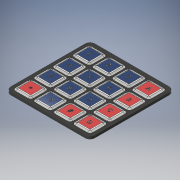
# Autodesk Inventor part: keypad
Saved by Autodesk Inventor 2019 (Build 230136000, 136)
## iProperties
Created: 2018-06-23
Part Number: keypad
Material: Generic
Document SubType Name: Modeling
Designer: Akshay
Density: 1 g/cm^3
Appearance: Default
Author: Akshay
Autodesk Inventor part; units mm, degrees
ref_plane "YZ Plane" through (0, 0, 0) normal (1, 0, 0) x (0, 1, 0)
ref_plane "XZ Plane" through (0, 0, 0) normal (0, 1, 0) x (-1, 0, 0)
ref_plane "XY Plane" through (0, 0, 0) normal (0, 0, 1) x (1, 0, 0)
sketch "Sketch1" plane through (0, 0, 0) normal (0, 1, 0) x (-1, 0, 0)
  line L0 (34, -34) -> (-34, -34)
  line L1 (-34, -34) -> (-34, 34)
  line L2 (-34, 34) -> (34, 34)
  line L3 (34, 34) -> (34, -34)
  line L4 (34, -34) -> (-34, 34) construction
  line L5 (-34, -34) -> (34, 34) construction
  point P0 (0, 0)
  dimension "d0" = 68
  dimension "d1" = 68
  constraints: 12 end point, 2 midpoint, 2 parallel, 1 horizontal, 1 perpendicular
  measures "d0" distance of L1.end L2.end
  measures "d1" distance of L0.end L1.end
extrude "Extrusion1" add sketch "Sketch1" along normal blind 2
fillet "Fillet1" radius 4 4 edges at (-34, 1, -34) (-34, 1, 34) (34, 1, 34) (34, 1, -34)
sketch "Sketch3" plane through (0, 2, 0) normal (0, 1, 0) x (1, 0, 0)
  line L0 (18, 29.4093) -> (30, 29.4093)
  line L1 (2, 29.4093) -> (14, 29.4093)
  line L2 (-30, 29.4093) -> (-18, 29.4093)
  line L3 (-14, 29.4093) -> (-2, 29.4093)
  line L4 (-30, 17.4093) -> (-30, 29.4093)
  line L5 (-18, 29.4093) -> (-18, 17.4093)
  line L6 (-14, 29.4093) -> (-14, 17.4093)
  line L7 (-18, 17.4093) -> (-30, 17.4093)
  line L8 (-2, 17.4093) -> (-14, 17.4093)
  line L9 (-2, 17.4093) -> (-2, 29.4093)
  line L10 (2, 29.4093) -> (2, 17.4093)
  line L11 (30, 17.4093) -> (18, 17.4093)
  line L12 (14, 17.4093) -> (2, 17.4093)
  line L13 (14, 17.4093) -> (14, 29.4093)
  line L14 (18, 29.4093) -> (18, 17.4093)
  line L15 (2, 13.4093) -> (14, 13.4093)
  line L16 (18, 13.4093) -> (30, 13.4093)
  line L17 (30, 1.9653) -> (18, 1.861)
  line L18 (18, 13.4093) -> (18, 1.861)
  line L19 (14, 1.8263) -> (14, 13.4093)
  line L20 (2, 13.4093) -> (2, 1.722)
  line L21 (-2, 1.6873) -> (-2, 13.4093)
  line L22 (-14, 13.4093) -> (-14, 1.5831)
  line L23 (-18, 13.4093) -> (-18, 1.5483)
  line L24 (-30, 1.4441) -> (-30, 13.4093)
  line L25 (-18, 1.5483) -> (-30, 1.4441)
  line L26 (-30, 13.4093) -> (-18, 13.4093)
  line L27 (-14, 13.4093) -> (-2, 13.4093)
  line L28 (14, 1.8263) -> (2, 1.722)
  line L29 (-2, 1.6873) -> (-14, 1.5831)
  line L30 (18, -2) -> (30, -2)
  line L31 (-30, -30) -> (-30, -18)
  line L32 (-30, -14) -> (-30, -2)
  line L33 (-18, -2) -> (-18, -14)
  line L34 (-18, -18) -> (-18, -30)
  line L35 (-30, -14) -> (-18, -14)
  line L36 (-30, -18) -> (-18, -18)
  line L37 (-14, -14) -> (-2, -14)
  line L38 (-14, -2) -> (-14, -14)
  line L39 (-14, -18) -> (-14, -30)
  line L40 (-2, -30) -> (-2, -18)
  line L41 (-2, -14) -> (-2, -2)
  line L42 (-14, -18) -> (-2, -18)
  line L43 (2, -14) -> (14, -14)
  line L44 (18, -14) -> (30, -14)
  line L45 (14, -30) -> (14, -18)
  line L46 (14, -14) -> (14, -2)
  line L47 (2, -2) -> (2, -14)
  line L48 (2, -18) -> (2, -30)
  line L49 (2, -18) -> (14, -18)
  line L50 (18, -18) -> (30, -18)
  line L51 (30, -30) -> (30, -18)
  line L52 (30, -14) -> (30, -2)
  line L53 (18, -2) -> (18, -14)
  line L54 (18, -18) -> (18, -30)
  line L55 (18, -30) -> (30, -30)
  line L56 (2, -30) -> (14, -30)
  line L57 (-30, -30) -> (-18, -30)
  line L58 (-14, -30) -> (-2, -30)
  line L59 (30, 1.9653) -> (30, 13.4093)
  line L60 (30, 17.4093) -> (30, 29.4093)
  line L61 (-30, -2) -> (-2, -2)
  line L62 (2, -2) -> (14, -2)
  point P0 (0, 0)
  point P1 (-34, -30)
  point P2 (-30, 34)
  constraints: 126 end point, 96 perpendicular, 4 horizontal, 2 point on line
extrude "Extrusion2" add sketch "Sketch3" along normal blind 1
fillet "Fillet2" radius 1 4 edges at (-30, 2.5, 18) (-18, 2.5, 18) (-30, 2.5, 30) (-18, 2.5, 30)
fillet "Fillet3" radius 1 4 edges at (-30, 2.5, 14) (-30, 2.5, 2) (-18, 2.5, 2) (-18, 2.5, 14)
fillet "Fillet4" radius 1 4 edges at (-18, 2.5, -1.5483) (-30, 2.5, -1.4441) (-18, 2.5, -13.4093) (-30, 2.5, -13.4093)
fillet "Fillet5" radius 1 4 edges at (-30, 2.5, -29.4093) (-18, 2.5, -29.4093) (-30, 2.5, -17.4093) (-18, 2.5, -17.4093)
fillet "Fillet6" radius 1 5 edges at (-14, 2.5, -17.4093) (-14, 2.5, -13.4093) (-14, 2.5, -29.4093) (-2, 2.5, -29.4093) (-2, 2.5, -17.4093)
fillet "Fillet7" radius 1 7 edges at (-2, 2.5, -13.4093) (-2, 2.5, -1.6873) (-14, 2.5, -1.5831) (-14, 2.5, 2) (-14, 2.5, 14) (-2, 2.5, 14) (-2, 2.5, 2)
fillet "Fillet8" radius 1 12 edges at (-2, 2.5, 18) (-2, 2.5, 30) (-14, 2.5, 30) (-14, 2.5, 18) (2, 2.5, 18) (2, 2.5, 30) (14, 2.5, 30) (14, 2.5, 18) (18, 2.5, 18) (30, 2.5, 30) (18, 2.5, 30) (30, 2.5, 18)
fillet "Fillet9" radius 1 8 edges at (2, 2.5, 2) (2, 2.5, 14) (14, 2.5, 14) (14, 2.5, 2) (18, 2.5, 14) (18, 2.5, 2) (30, 2.5, 2) (30, 2.5, 14)
fillet "Fillet10" radius 1 16 edges at (2, 2.5, -13.4093) (2, 2.5, -1.722) (14, 2.5, -1.8263) (14, 2.5, -13.4093) (18, 2.5, -13.4093) (18, 2.5, -1.861) (30, 2.5, -1.9653) (30, 2.5, -13.4093) (30, 2.5, -17.4093) (30, 2.5, -29.4093) (18, 2.5, -17.4093) (18, 2.5, -29.4093) (14, 2.5, -29.4093) (14, 2.5, -17.4093) (2, 2.5, -17.4093) (2, 2.5, -29.4093)
fillet "Fillet11" radius 1 8 edges at (-29.7071, 3, -17.7022) (-24, 3, -17.4093) (-18.2929, 3, -17.7022) (-18, 3, -23.4093) (-18.2929, 3, -29.1164) (-24, 3, -29.4093) (-29.7071, 3, -29.1164) (-30, 3, -23.4093)
fillet "Fillet12" radius 1 120 edges at (-13.7071, 3, -17.7022) (-8, 3, -17.4093) (-2.2929, 3, -17.7022) (-2, 3, -23.4093) (-2.2929, 3, -29.1164) (-8, 3, -29.4093) (-13.7071, 3, -29.1164) (-14, 3, -23.4093) (-13.704, 3, -1.8816) (-7.9913, 3, -1.6352) (-2.2898, 3, -1.9746) (-2, 3, -7.544) (-2.2929, 3, -13.1164) (-8, 3, -13.4093) (-13.7071, 3, -13.1164) (-14, 3, -7.5006) (-29.704, 3, -1.7426) (-23.9913, 3, -1.4963) (-18.2898, 3, -1.8356) (-18, 3, -7.4745) (-18.2929, 3, -13.1164) (-24, 3, -13.4093) (-29.7071, 3, -13.1164) (-30, 3, -7.4311) (2.296, 3, -2.0206) (8.0087, 3, -1.7742) (13.7102, 3, -2.1136) (14, 3, -7.6135) (13.7071, 3, -13.1164) (8, 3, -13.4093) (2.2929, 3, -13.1164) (2, 3, -7.57) (2.2929, 3, -17.7022) (8, 3, -17.4093) (13.7071, 3, -17.7022) (14, 3, -23.4093) (13.7071, 3, -29.1164) (8, 3, -29.4093) (2.2929, 3, -29.1164) (2, 3, -23.4093) (18.296, 3, -2.1596) (24.0087, 3, -1.9132) (29.7102, 3, -2.2526) (30, 3, -7.683) (29.7071, 3, -13.1164) (24, 3, -13.4093) (18.2929, 3, -13.1164) (18, 3, -7.6395) (18.2929, 3, -17.7022) (24, 3, -17.4093) (29.7071, 3, -17.7022) (30, 3, -23.4093) (29.7071, 3, -29.1164) (24, 3, -29.4093) (18.2929, 3, -29.1164) (18, 3, -23.4093) (18.2929, 3, 13.7071) (24, 3, 14) (29.7071, 3, 13.7071) (30, 3, 8) (29.7071, 3, 2.2929) (24, 3, 2) (18.2929, 3, 2.2929) (18, 3, 8) (18.2929, 3, 29.7071) (24, 3, 30) (29.7071, 3, 29.7071) (30, 3, 24) (29.7071, 3, 18.2929) (24, 3, 18) (18.2929, 3, 18.2929) (18, 3, 24) (2.2929, 3, 29.7071) (8, 3, 30) (13.7071, 3, 29.7071) (14, 3, 24) (13.7071, 3, 18.2929) (8, 3, 18) (2.2929, 3, 18.2929) (2, 3, 24) (2.2929, 3, 13.7071) (8, 3, 14) (13.7071, 3, 13.7071) (14, 3, 8) (13.7071, 3, 2.2929) (8, 3, 2) (2.2929, 3, 2.2929) (2, 3, 8) (-13.7071, 3, 29.7071) (-8, 3, 30) (-2.2929, 3, 29.7071) (-2, 3, 24) (-2.2929, 3, 18.2929) (-8, 3, 18) (-13.7071, 3, 18.2929) (-14, 3, 24) (-13.7071, 3, 13.7071) (-8, 3, 14) (-2.2929, 3, 13.7071) (-2, 3, 8) (-2.2929, 3, 2.2929) (-8, 3, 2) (-13.7071, 3, 2.2929) (-14, 3, 8) (-29.7071, 3, 13.7071) (-24, 3, 14) (-18.2929, 3, 13.7071) (-18, 3, 8) (-18.2929, 3, 2.2929) (-24, 3, 2) (-29.7071, 3, 2.2929) (-30, 3, 8) (-29.7071, 3, 29.7071) (-24, 3, 30) (-18.2929, 3, 29.7071) (-18, 3, 24) (-18.2929, 3, 18.2929) (-24, 3, 18) (-29.7071, 3, 18.2929) (-30, 3, 24)
fillet "Fillet13" radius 2 256 edges at (24, 2, 14) (24, 2.0005, 14) (29.7071, 2, 13.7071) (29.7071, 2.0005, 13.7071) (30, 2, 8) (30, 2.0005, 8) (29.7071, 2, 2.2929) (29.7071, 2.0005, 2.2929) (24, 2, 2) (24, 2.0005, 2) (18.2929, 2, 2.2929) (18.2929, 2.0005, 2.2929) (18, 2, 8) (18, 2.0005, 8) (18.2929, 2, 13.7071) (18.2929, 2.0005, 13.7071) (13.7071, 2, 13.7071) (13.7071, 2.0005, 13.7071) (8, 2, 14) (8, 2.0005, 14) (2.2929, 2, 13.7071) (2.2929, 2.0005, 13.7071) (2, 2, 8) (2, 2.0005, 8) (2.2929, 2, 2.2929) (2.2929, 2.0005, 2.2929) (8, 2, 2) (8, 2.0005, 2) (13.7071, 2, 2.2929) (13.7071, 2.0005, 2.2929) (14, 2, 8) (14, 2.0005, 8) (13.7071, 2, 29.7071) (13.7071, 2.0005, 29.7071) (8, 2, 30) (8, 2.0005, 30) (2.2929, 2, 29.7071) (2.2929, 2.0005, 29.7071) (2, 2, 24) (2, 2.0005, 24) (2.2929, 2, 18.2929) (2.2929, 2.0005, 18.2929) (8, 2, 18) (8, 2.0005, 18) (13.7071, 2, 18.2929) (13.7071, 2.0005, 18.2929) (14, 2, 24) (14, 2.0005, 24) (18.2929, 2, 18.2929) (18.2929, 2.0005, 18.2929) (24, 2, 18) (24, 2.0005, 18) (29.7071, 2, 18.2929) (29.7071, 2.0005, 18.2929) (30, 2, 24) (30, 2.0005, 24) (29.7071, 2, 29.7071) (29.7071, 2.0005, 29.7071) (24, 2, 30) (24, 2.0005, 30) (18.2929, 2, 29.7071) (18.2929, 2.0005, 29.7071) (18, 2, 24) (18, 2.0005, 24) (29.7102, 2, -2.2526) (29.7102, 2.0005, -2.2526) (24.0087, 2, -1.9132) (24.0087, 2.0005, -1.9132) (18.296, 2, -2.1596) (18.296, 2.0005, -2.1596) (18, 2, -7.6395) (18, 2.0005, -7.6395) (18.2929, 2, -13.1164) (18.2929, 2.0005, -13.1164) (24, 2, -13.4093) (24, 2.0005, -13.4093) (29.7071, 2, -13.1164) (29.7071, 2.0005, -13.1164) (30, 2, -7.683) (30, 2.0005, -7.683) (13.7102, 2, -2.1136) (13.7102, 2.0005, -2.1136) (8.0087, 2, -1.7742) (8.0087, 2.0005, -1.7742) (2.296, 2, -2.0206) (2.296, 2.0005, -2.0206) (2, 2, -7.57) (2, 2.0005, -7.57) (2.2929, 2, -13.1164) (2.2929, 2.0005, -13.1164) (8, 2, -13.4093) (8, 2.0005, -13.4093) (13.7071, 2, -13.1164) (13.7071, 2.0005, -13.1164) (14, 2, -7.6135) (14, 2.0005, -7.6135) (18.2929, 2, -29.1164) (18.2929, 2.0005, -29.1164) (24, 2, -29.4093) (24, 2.0005, -29.4093) (29.7071, 2, -29.1164) (29.7071, 2.0005, -29.1164) (30, 2.0005, -23.4093) (30, 2, -23.4093) (29.7071, 2.0005, -17.7022) (29.7071, 2, -17.7022) (24, 2, -17.4093) (24, 2.0005, -17.4093) (18.2929, 2, -17.7022) (18.2929, 2.0005, -17.7022) (18, 2, -23.4093) (18, 2.0005, -23.4093) (13.7071, 2, -17.7022) (13.7071, 2.0005, -17.7022) (8, 2, -17.4093) (8, 2.0005, -17.4093) (2.2929, 2, -17.7022) (2.2929, 2.0005, -17.7022) (2, 2, -23.4093) (2, 2.0005, -23.4093) (2.2929, 2, -29.1164) (2.2929, 2.0005, -29.1164) (8, 2, -29.4093) (8, 2.0005, -29.4093) (13.7071, 2, -29.1164) (13.7071, 2.0005, -29.1164) (14, 2, -23.4093) (14, 2.0005, -23.4093) (-2.2929, 2, -17.7022) (-2.2929, 2.0005, -17.7022) (-8, 2, -17.4093) (-8, 2.0005, -17.4093) (-13.7071, 2, -17.7022) (-13.7071, 2.0005, -17.7022) (-14, 2, -23.4093) (-14, 2.0005, -23.4093) (-13.7071, 2, -29.1164) (-13.7071, 2.0005, -29.1164) (-8, 2, -29.4093) (-8, 2.0005, -29.4093) (-2.2929, 2, -29.1164) (-2.2929, 2.0005, -29.1164) (-2, 2, -23.4093) (-2, 2.0005, -23.4093) (-2.2898, 2, -1.9746) (-2.2898, 2.0005, -1.9746) (-7.9913, 2, -1.6352) (-7.9913, 2.0005, -1.6352) (-13.704, 2, -1.8816) (-13.704, 2.0005, -1.8816) (-14, 2, -7.5006) (-14, 2.0005, -7.5006) (-13.7071, 2, -13.1164) (-13.7071, 2.0005, -13.1164) (-8, 2, -13.4093) (-8, 2.0005, -13.4093) (-2.2929, 2, -13.1164) (-2.2929, 2.0005, -13.1164) (-2, 2, -7.544) (-2, 2.0005, -7.544) (-2.2929, 2, 13.7071) (-2.2929, 2.0005, 13.7071) (-8, 2, 14) (-8, 2.0005, 14) (-13.7071, 2, 13.7071) (-13.7071, 2.0005, 13.7071) (-14, 2, 8) (-14, 2.0005, 8) (-13.7071, 2, 2.2929) (-13.7071, 2.0005, 2.2929) (-8, 2, 2) (-8, 2.0005, 2) (-2.2929, 2, 2.2929) (-2.2929, 2.0005, 2.2929) (-2, 2, 8) (-2, 2.0005, 8) (-2.2929, 2, 29.7071) (-2.2929, 2.0005, 29.7071) (-8, 2, 30) (-8, 2.0005, 30) (-13.7071, 2, 29.7071) (-13.7071, 2.0005, 29.7071) (-14, 2, 24) (-14, 2.0005, 24) (-13.7071, 2, 18.2929) (-13.7071, 2.0005, 18.2929) (-8, 2, 18) (-8, 2.0005, 18) (-2.2929, 2, 18.2929) (-2.2929, 2.0005, 18.2929) (-2, 2, 24) (-2, 2.0005, 24) (-18.2929, 2, 29.7071) (-18.2929, 2.0005, 29.7071) (-24, 2, 30) (-24, 2.0005, 30) (-29.7071, 2, 29.7071) (-29.7071, 2.0005, 29.7071) (-30, 2, 24) (-30, 2.0005, 24) (-29.7071, 2, 18.2929) (-29.7071, 2.0005, 18.2929) (-24, 2, 18) (-24, 2.0005, 18) (-18.2929, 2, 18.2929) (-18.2929, 2.0005, 18.2929) (-18, 2, 24) (-18, 2.0005, 24) (-18.2929, 2, 13.7071) (-18.2929, 2.0005, 13.7071) (-24, 2, 14) (-24, 2.0005, 14) (-29.7071, 2, 13.7071) (-29.7071, 2.0005, 13.7071) (-30, 2, 8) (-30, 2.0005, 8) (-29.7071, 2, 2.2929) (-29.7071, 2.0005, 2.2929) (-24, 2, 2) (-24, 2.0005, 2) (-18.2929, 2, 2.2929) (-18.2929, 2.0005, 2.2929) (-18, 2, 8) (-18, 2.0005, 8) (-18.2898, 2, -1.8356) (-18.2898, 2.0005, -1.8356) (-23.9913, 2, -1.4963) (-23.9913, 2.0005, -1.4963) (-29.704, 2, -1.7426) (-29.704, 2.0005, -1.7426) (-30, 2, -7.4311) (-30, 2.0005, -7.4311) (-29.7071, 2, -13.1164) (-29.7071, 2.0005, -13.1164) (-24, 2, -13.4093) (-24, 2.0005, -13.4093) (-18.2929, 2, -13.1164) (-18.2929, 2.0005, -13.1164) (-18, 2, -7.4745) (-18, 2.0005, -7.4745) (-18.2929, 2, -17.7022) (-18.2929, 2.0005, -17.7022) (-24, 2, -17.4093) (-24, 2.0005, -17.4093) (-29.7071, 2, -17.7022) (-29.7071, 2.0005, -17.7022) (-30, 2, -23.4093) (-30, 2.0005, -23.4093) (-29.7071, 2, -29.1164) (-29.7071, 2.0005, -29.1164) (-24, 2, -29.4093) (-24, 2.0005, -29.4093) (-18.2929, 2, -29.1164) (-18.2929, 2.0005, -29.1164) (-18, 2, -23.4093) (-18, 2.0005, -23.4093)
sketch "Sketch4" plane through (0, 3, 0) normal (0, 1, 0) x (1, 0, 0)
  line L0 (-25.4936, 25.6237) -> (-19.6405, 25.6237) construction
  line L1 (-19.6405, 25.6237) -> (-19.6405, 19.1202) construction
  line L2 (-19.6405, 19.1202) -> (-25.4936, 19.1202) construction
  line L3 (-25.4936, 19.1202) -> (-25.4936, 25.6237) construction
  line L4 (-9.6251, 25.2335) -> (-7.3379, 25.2335) construction
  line L5 (-7.3379, 25.2335) -> (-7.3379, 22.1213) construction
  line L6 (-7.3379, 22.1213) -> (-9.6251, 22.1213) construction
  line L7 (-9.6251, 22.1213) -> (-9.6251, 25.2335) construction
  line L8 (6.3734, 24.9733) -> (8.6606, 24.9733) construction
  line L9 (8.6606, 24.9733) -> (8.6606, 21.7969) construction
  line L10 (8.6606, 21.7969) -> (6.3734, 21.7969) construction
  line L11 (6.3734, 21.7969) -> (6.3734, 24.9733) construction
  line L12 (-24.9733, 8.9748) -> (-22.426, 8.9748) construction
  line L13 (-22.426, 8.9748) -> (-22.426, 5.9268) construction
  line L14 (-22.426, 5.9268) -> (-24.9733, 5.9268) construction
  line L15 (-24.9733, 5.9268) -> (-24.9733, 8.9748) construction
  line L16 (-8.9748, 8.8447) -> (-6.6876, 8.8447) construction
  line L17 (-6.6876, 8.8447) -> (-6.6876, 5.7325) construction
  line L18 (-6.6876, 5.7325) -> (-8.9748, 5.7325) construction
  line L19 (-8.9748, 5.7325) -> (-8.9748, 8.8447) construction
  line L20 (6.7636, 9.365) -> (9.0508, 9.365) construction
  line L21 (9.0508, 9.365) -> (9.0508, 6.196) construction
  line L22 (9.0508, 6.196) -> (6.7636, 6.196) construction
  line L23 (6.7636, 6.196) -> (6.7636, 9.365) construction
  line L24 (-25.4395, -6.3515) -> (-23.1523, -6.3515) construction
  line L25 (-23.1523, -6.3515) -> (-23.1523, -9.3995) construction
  line L26 (-23.1523, -9.3995) -> (-25.4395, -9.3995) construction
  line L27 (-25.4395, -9.3995) -> (-25.4395, -6.3515) construction
  line L28 (-9.2349, -6.6335) -> (-6.9477, -6.6335) construction
  line L29 (-6.9477, -6.6335) -> (-6.9477, -9.8199) construction
  line L30 (-6.9477, -9.8199) -> (-9.2349, -9.8199) construction
  line L31 (-9.2349, -9.8199) -> (-9.2349, -6.6335) construction
  line L32 (6.8094, -6.4337) -> (8.9208, -6.4337) construction
  line L33 (8.9208, -6.4337) -> (8.9208, -9.6027) construction
  line L34 (8.9208, -9.6027) -> (6.8094, -9.6027) construction
  line L35 (6.8094, -9.6027) -> (6.8094, -6.4337) construction
  line L36 (-8.7057, -22.502) -> (-6.4185, -22.502) construction
  line L37 (-6.4185, -22.502) -> (-6.4185, -25.676) construction
  line L38 (-6.4185, -25.676) -> (-8.7057, -25.676) construction
  line L39 (-8.7057, -25.676) -> (-8.7057, -22.502) construction
  line L40 (23.0223, 24.8433) -> (25.5763, 24.8433) construction
  line L41 (25.5763, 24.8433) -> (25.5763, 21.7953) construction
  line L42 (25.5763, 21.7953) -> (23.0223, 21.7953) construction
  line L43 (23.0223, 21.7953) -> (23.0223, 24.8433) construction
  line L44 (22.7622, 9.2349) -> (26.2727, 9.2349) construction
  line L45 (26.2727, 9.2349) -> (26.2727, 6.1869) construction
  line L46 (26.2727, 6.1869) -> (22.7622, 6.1869) construction
  line L47 (22.7622, 6.1869) -> (22.7622, 9.2349) construction
  line L48 (22.3719, -5.9832) -> (24.8889, -5.9832) construction
  line L49 (24.8889, -5.9832) -> (24.8889, -9.1399) construction
  line L50 (24.8889, -9.1399) -> (22.3719, -9.1399) construction
  line L51 (22.3719, -9.1399) -> (22.3719, -5.9832) construction
  line L52 (22.3719, -22.502) -> (25.2149, -22.502) construction
  line L53 (25.2149, -22.502) -> (25.2149, -25.55) construction
  line L54 (25.2149, -25.55) -> (22.3719, -25.55) construction
  line L55 (22.3719, -25.55) -> (22.3719, -22.502) construction
  line L56 (-25.1536, -22.9863) -> (-22.8664, -22.9863) construction
  line L57 (-22.8664, -22.9863) -> (-22.8664, -24.8808) construction
  line L58 (-22.8664, -24.8808) -> (-25.1536, -24.8808) construction
  line L59 (-25.1536, -24.8808) -> (-25.1536, -22.9863) construction
  line L60 (6.5254, -22.296) -> (9.5758, -22.296) construction
  line L61 (9.5758, -22.296) -> (9.5758, -25.344) construction
  line L62 (9.5758, -25.344) -> (6.5254, -25.344) construction
  line L63 (6.5254, -25.344) -> (6.5254, -22.296) construction
  line L64 (23.0025, 21.7953) -> (24.0301, 24.8433)
  line L65 (24.0301, 24.8433) -> (24.529, 24.8433)
  line L66 (24.529, 24.8433) -> (25.5565, 21.7953)
  line L67 (25.5565, 21.7953) -> (25.1292, 21.7953)
  line L68 (25.1292, 21.7953) -> (24.8526, 22.6474)
  line L69 (24.8526, 22.6474) -> (23.6892, 22.6474)
  line L70 (23.6892, 22.6474) -> (23.4126, 21.7953)
  line L71 (23.4126, 21.7953) -> (23.0025, 21.7953)
  line L72 (24.7414, 22.9932) -> (24.2697, 24.4283)
  line L73 (24.2697, 24.4283) -> (23.8004, 22.9932)
  line L74 (23.8004, 22.9932) -> (24.7414, 22.9932)
  spline S0 degree 2 poles (7.4182, 24.6201) (7.3071, 24.6201) (7.0872, 24.5658) (6.981, 24.5238) knots 0 0 0 1 2 2 2
  spline S1 degree 2 poles (6.981, 24.5238) (6.8822, 24.4818) (6.7365, 24.3929) (6.6797, 24.3534) knots 0 0 0 1 2 2 2
  line L75 (6.6797, 24.3534) -> (6.655, 24.3534)
  line L76 (6.655, 24.3534) -> (6.655, 24.7856)
  spline S2 degree 2 poles (6.655, 24.7856) (6.7884, 24.8573) (7.2453, 24.9733) (7.4503, 24.9733) knots 0 0 0 1 2 2 2
  spline S3 degree 2 poles (7.4503, 24.9733) (7.6578, 24.9733) (7.9666, 24.8894) (8.0925, 24.8004) knots 0 0 0 1 2 2 2
  spline S4 degree 2 poles (8.0925, 24.8004) (8.2259, 24.7041) (8.3642, 24.425) (8.3642, 24.2373) knots 0 0 0 1 2 2 2
  spline S5 degree 2 poles (8.3642, 24.2373) (8.3642, 23.9853) (8.0333, 23.605) (7.8011, 23.5556) knots 0 0 0 1 2 2 2
  line L77 (7.8011, 23.5556) -> (7.8011, 23.5259)
  spline S6 degree 2 poles (7.8011, 23.5259) (7.8974, 23.5062) (8.1172, 23.4172) (8.2111, 23.3283) knots 0 0 0 1 2 2 2
  spline S7 degree 2 poles (8.2111, 23.3283) (8.305, 23.2419) (8.4235, 22.9652) (8.4235, 22.7651) knots 0 0 0 1 2 2 2
  spline S8 degree 2 poles (8.4235, 22.7651) (8.4235, 22.5601) (8.2827, 22.2119) (8.1543, 22.0785) knots 0 0 0 1 2 2 2
  spline S9 degree 2 poles (8.1543, 22.0785) (8.0209, 21.9402) (7.643, 21.7969) (7.4034, 21.7969) knots 0 0 0 1 2 2 2
  spline S10 degree 2 poles (7.4034, 21.7969) (7.1737, 21.7969) (6.7241, 21.9081) (6.571, 21.9846) knots 0 0 0 1 2 2 2
  line L78 (6.571, 21.9846) -> (6.571, 22.4169)
  line L79 (6.571, 22.4169) -> (6.6006, 22.4169)
  spline S11 degree 2 poles (6.6006, 22.4169) (6.7291, 22.323) (7.1638, 22.1501) (7.3787, 22.1501) knots 0 0 0 1 2 2 2
  spline S12 degree 2 poles (7.3787, 22.1501) (7.5047, 22.1501) (7.7566, 22.2292) (7.8406, 22.3205) knots 0 0 0 1 2 2 2
  spline S13 degree 2 poles (7.8406, 22.3205) (7.9221, 22.4119) (8.0086, 22.6293) (8.0086, 22.7948) knots 0 0 0 1 2 2 2
  spline S14 degree 2 poles (8.0086, 22.7948) (8.0086, 22.9603) (7.9122, 23.1752) (7.8258, 23.2369) knots 0 0 0 1 2 2 2
  spline S15 degree 2 poles (7.8258, 23.2369) (7.7393, 23.2987) (7.5047, 23.3456) (7.3664, 23.3456) knots 0 0 0 1 2 2 2
  line L80 (7.3664, 23.3456) -> (7.1934, 23.3456)
  line L81 (7.1934, 23.3456) -> (7.1934, 23.684)
  line L82 (7.1934, 23.684) -> (7.3293, 23.684)
  spline S16 degree 2 poles (7.3293, 23.684) (7.6035, 23.684) (7.9493, 23.9458) (7.9493, 24.1953) knots 0 0 0 1 2 2 2
  spline S17 degree 2 poles (7.9493, 24.1953) (7.9493, 24.3114) (7.8604, 24.4769) (7.7887, 24.5263) knots 0 0 0 1 2 2 2
  spline S18 degree 2 poles (7.7887, 24.5263) (7.7122, 24.5781) (7.5244, 24.6201) (7.4182, 24.6201) knots 0 0 0 1 2 2 2
  line L83 (-7.5232, 22.1213) -> (-9.4028, 22.1213)
  line L84 (-9.4028, 22.1213) -> (-9.4028, 22.5535)
  spline S19 degree 2 poles (-9.4028, 22.5535) (-9.2003, 22.7437) (-8.8397, 23.0969) (-8.6668, 23.2871) knots 0 0 0 1 2 2 2
  spline S20 degree 2 poles (-8.6668, 23.2871) (-8.3185, 23.67) (-8.0641, 24.1294) (-8.0641, 24.3739) knots 0 0 0 1 2 2 2
  spline S21 degree 2 poles (-8.0641, 24.3739) (-8.0641, 24.5024) (-8.1431, 24.695) (-8.2148, 24.7568) knots 0 0 0 1 2 2 2
  spline S22 degree 2 poles (-8.2148, 24.7568) (-8.2864, 24.8185) (-8.4741, 24.8803) (-8.5877, 24.8803) knots 0 0 0 1 2 2 2
  spline S23 degree 2 poles (-8.5877, 24.8803) (-8.6964, 24.8803) (-8.9187, 24.8259) (-9.02, 24.7839) knots 0 0 0 1 2 2 2
  spline S24 degree 2 poles (-9.02, 24.7839) (-9.1064, 24.7494) (-9.267, 24.6506) (-9.3164, 24.616) knots 0 0 0 1 2 2 2
  line L85 (-9.3164, 24.616) -> (-9.3386, 24.616)
  line L86 (-9.3386, 24.616) -> (-9.3386, 25.0507)
  spline S25 degree 2 poles (-9.3386, 25.0507) (-9.2126, 25.1125) (-8.7606, 25.2335) (-8.5581, 25.2335) knots 0 0 0 1 2 2 2
  spline S26 degree 2 poles (-8.5581, 25.2335) (-8.1308, 25.2335) (-7.6491, 24.7815) (-7.6491, 24.3961) knots 0 0 0 1 2 2 2
  spline S27 degree 2 poles (-7.6491, 24.3961) (-7.6491, 24.2158) (-7.7331, 23.9145) (-7.8072, 23.7861) knots 0 0 0 1 2 2 2
  spline S28 degree 2 poles (-7.8072, 23.7861) (-7.8813, 23.6527) (-8.0962, 23.3908) (-8.2148, 23.2649) knots 0 0 0 1 2 2 2
  spline S29 degree 2 poles (-8.2148, 23.2649) (-8.4074, 23.0549) (-8.8792, 22.6054) (-9.02, 22.4745) knots 0 0 0 1 2 2 2
  line L87 (-9.02, 22.4745) -> (-7.5232, 22.4745)
  line L88 (-7.5232, 22.4745) -> (-7.5232, 22.1213)
  line L89 (-23.5448, 22.5658) -> (-25.0317, 22.5658)
  line L90 (-25.0317, 22.5658) -> (-25.0317, 22.877)
  line L91 (-25.0317, 22.877) -> (-24.4784, 22.877)
  line L92 (-24.4784, 22.877) -> (-24.4784, 24.9197)
  line L93 (-24.4784, 24.9197) -> (-25.0317, 24.9197)
  line L94 (-25.0317, 24.9197) -> (-25.0317, 25.1988)
  spline S30 degree 2 poles (-25.0317, 25.1988) (-24.718, 25.1988) (-24.4216, 25.3767) (-24.4019, 25.6237) knots 0 0 0 1 2 2 2
  line L95 (-24.4019, 25.6237) -> (-24.0857, 25.6237)
  line L96 (-24.0857, 25.6237) -> (-24.0857, 22.877)
  line L97 (-24.0857, 22.877) -> (-23.5448, 22.877)
  line L98 (-23.5448, 22.877) -> (-23.5448, 22.5658)
  line L99 (-22.7898, 6.9741) -> (-23.1529, 6.9741)
  line L100 (-23.1529, 6.9741) -> (-23.1529, 5.9268)
  line L101 (-23.1529, 5.9268) -> (-23.5457, 5.9268)
  line L102 (-23.5457, 5.9268) -> (-23.5457, 6.9741)
  line L103 (-23.5457, 6.9741) -> (-24.8918, 6.9741)
  line L104 (-24.8918, 6.9741) -> (-24.8918, 7.4039)
  line L105 (-24.8918, 7.4039) -> (-23.5284, 8.9748)
  line L106 (-23.5284, 8.9748) -> (-23.1529, 8.9748)
  line L107 (-23.1529, 8.9748) -> (-23.1529, 7.3026)
  line L108 (-23.1529, 7.3026) -> (-22.7898, 7.3026)
  line L109 (-22.7898, 7.3026) -> (-22.7898, 6.9741)
  line L110 (-23.5457, 7.3026) -> (-23.5457, 8.4931)
  line L111 (-23.5457, 8.4931) -> (-24.5707, 7.3026)
  line L112 (-24.5707, 7.3026) -> (-23.5457, 7.3026)
  line L113 (-23.303, -6.8085) -> (-24.622, -9.3995)
  line L114 (-24.622, -9.3995) -> (-25.0567, -9.3995)
  line L115 (-25.0567, -9.3995) -> (-23.6636, -6.7097)
  line L116 (-23.6636, -6.7097) -> (-25.237, -6.7097)
  line L117 (-25.237, -6.7097) -> (-25.237, -6.3515)
  line L118 (-25.237, -6.3515) -> (-23.303, -6.3515)
  line L119 (-23.303, -6.3515) -> (-23.303, -6.8085)
  line L120 (-23.0911, -24.3547) -> (-23.2245, -24.5795)
  line L121 (-23.2245, -24.5795) -> (-23.8939, -24.1349)
  line L122 (-23.8939, -24.1349) -> (-23.8791, -24.8808)
  line L123 (-23.8791, -24.8808) -> (-24.1359, -24.8808)
  line L124 (-24.1359, -24.8808) -> (-24.1236, -24.1349)
  line L125 (-24.1236, -24.1349) -> (-24.788, -24.582)
  line L126 (-24.788, -24.582) -> (-24.9239, -24.3572)
  line L127 (-24.9239, -24.3572) -> (-24.2002, -23.9324)
  line L128 (-24.2002, -23.9324) -> (-24.9239, -23.51)
  line L129 (-24.9239, -23.51) -> (-24.788, -23.2852)
  line L130 (-24.788, -23.2852) -> (-24.1211, -23.7323)
  line L131 (-24.1211, -23.7323) -> (-24.1359, -22.9863)
  line L132 (-24.1359, -22.9863) -> (-23.8791, -22.9863)
  line L133 (-23.8791, -22.9863) -> (-23.8964, -23.7323)
  line L134 (-23.8964, -23.7323) -> (-23.2245, -23.2877)
  line L135 (-23.2245, -23.2877) -> (-23.0911, -23.5125)
  line L136 (-23.0911, -23.5125) -> (-23.8148, -23.9324)
  line L137 (-23.8148, -23.9324) -> (-23.0911, -24.3547)
  spline S31 degree 2 poles (-6.9049, 6.765) (-6.9049, 6.5451) (-7.0457, 6.1697) (-7.1742, 6.0314) knots 0 0 0 1 2 2 2
  spline S32 degree 2 poles (-7.1742, 6.0314) (-7.3026, 5.8931) (-7.6854, 5.7325) (-7.9226, 5.7325) knots 0 0 0 1 2 2 2
  spline S33 degree 2 poles (-7.9226, 5.7325) (-8.1399, 5.7325) (-8.5648, 5.8288) (-8.7204, 5.9054) knots 0 0 0 1 2 2 2
  line L138 (-8.7204, 5.9054) -> (-8.7204, 6.3377)
  line L139 (-8.7204, 6.3377) -> (-8.6907, 6.3377)
  spline S34 degree 2 poles (-8.6907, 6.3377) (-8.6438, 6.3031) (-8.4684, 6.2142) (-8.3622, 6.1746) knots 0 0 0 1 2 2 2
  spline S35 degree 2 poles (-8.3622, 6.1746) (-8.2412, 6.1326) (-8.0411, 6.0857) (-7.9152, 6.0857) knots 0 0 0 1 2 2 2
  spline S36 degree 2 poles (-7.9152, 6.0857) (-7.7917, 6.0857) (-7.5595, 6.1746) (-7.4755, 6.271) knots 0 0 0 1 2 2 2
  spline S37 degree 2 poles (-7.4755, 6.271) (-7.3989, 6.3624) (-7.3199, 6.6044) (-7.3199, 6.7674) knots 0 0 0 1 2 2 2
  spline S38 degree 2 poles (-7.3199, 6.7674) (-7.3199, 6.9305) (-7.4088, 7.1379) (-7.4928, 7.2071) knots 0 0 0 1 2 2 2
  spline S39 degree 2 poles (-7.4928, 7.2071) (-7.5792, 7.2837) (-7.8361, 7.3479) (-7.9917, 7.3479) knots 0 0 0 1 2 2 2
  spline S40 degree 2 poles (-7.9917, 7.3479) (-8.1597, 7.3479) (-8.4931, 7.296) (-8.5944, 7.2738) knots 0 0 0 1 2 2 2
  line L140 (-8.5944, 7.2738) -> (-8.5944, 8.8447)
  line L141 (-8.5944, 8.8447) -> (-6.9222, 8.8447)
  line L142 (-6.9222, 8.8447) -> (-6.9222, 8.4866)
  line L143 (-6.9222, 8.4866) -> (-8.2017, 8.4866)
  line L144 (-8.2017, 8.4866) -> (-8.2017, 7.6739)
  spline S41 degree 2 poles (-8.2017, 7.6739) (-8.1276, 7.6838) (-7.9843, 7.6912) (-7.925, 7.6912) knots 0 0 0 1 2 2 2
  spline S42 degree 2 poles (-7.925, 7.6912) (-7.6904, 7.6912) (-7.3668, 7.6147) (-7.2186, 7.501) knots 0 0 0 1 2 2 2
  spline S43 degree 2 poles (-7.2186, 7.501) (-7.0679, 7.3874) (-6.9049, 7.0416) (-6.9049, 6.765) knots 0 0 0 1 2 2 2
  spline S44 degree 2 poles (-8.0913, -9.8199) (-8.3186, -9.8199) (-8.6915, -9.684) (-8.8224, -9.558) knots 0 0 0 1 2 2 2
  spline S45 degree 2 poles (-8.8224, -9.558) (-8.9509, -9.4345) (-9.0843, -9.0986) (-9.0843, -8.9084) knots 0 0 0 1 2 2 2
  spline S46 degree 2 poles (-9.0843, -8.9084) (-9.0843, -8.6614) (-8.82, -8.2465) (-8.568, -8.123) knots 0 0 0 1 2 2 2
  line L145 (-8.568, -8.123) -> (-8.568, -8.1106)
  spline S47 degree 2 poles (-8.568, -8.1106) (-8.7928, -7.9797) (-9.0102, -7.6685) (-9.0102, -7.4363) knots 0 0 0 1 2 2 2
  spline S48 degree 2 poles (-9.0102, -7.4363) (-9.0102, -7.093) (-8.4915, -6.6335) (-8.0913, -6.6335) knots 0 0 0 1 2 2 2
  spline S49 degree 2 poles (-8.0913, -6.6335) (-7.6764, -6.6335) (-7.1749, -7.0683) (-7.1749, -7.4091) knots 0 0 0 1 2 2 2
  spline S50 degree 2 poles (-7.1749, -7.4091) (-7.1749, -7.6141) (-7.4145, -8.0143) (-7.6393, -8.1279) knots 0 0 0 1 2 2 2
  line L146 (-7.6393, -8.1279) -> (-7.6393, -8.1403)
  spline S51 degree 2 poles (-7.6393, -8.1403) (-7.3725, -8.2638) (-7.0984, -8.6194) (-7.0984, -8.901) knots 0 0 0 1 2 2 2
  spline S52 degree 2 poles (-7.0984, -8.901) (-7.0984, -9.2913) (-7.6665, -9.8199) (-8.0913, -9.8199) knots 0 0 0 1 2 2 2
  spline S53 degree 2 poles (-7.5183, -8.9405) (-7.5183, -8.7528) (-7.6665, -8.5305) (-7.8764, -8.4169) knots 0 0 0 1 2 2 2
  spline S54 degree 2 poles (-7.8764, -8.4169) (-7.9456, -8.3774) (-8.1778, -8.286) (-8.3235, -8.2267) knots 0 0 0 1 2 2 2
  spline S55 degree 2 poles (-8.3235, -8.2267) (-8.4915, -8.3379) (-8.6718, -8.6688) (-8.6718, -8.8788) knots 0 0 0 1 2 2 2
  spline S56 degree 2 poles (-8.6718, -8.8788) (-8.6718, -9.1554) (-8.3383, -9.5161) (-8.0864, -9.5161) knots 0 0 0 1 2 2 2
  spline S57 degree 2 poles (-8.0864, -9.5161) (-7.8295, -9.5161) (-7.5183, -9.2073) (-7.5183, -8.9405) knots 0 0 0 1 2 2 2
  spline S58 degree 2 poles (-7.5751, -7.4141) (-7.5751, -7.2091) (-7.8493, -6.9349) (-8.0938, -6.9349) knots 0 0 0 1 2 2 2
  spline S59 degree 2 poles (-8.0938, -6.9349) (-8.3161, -6.9349) (-8.6001, -7.1794) (-8.6001, -7.3894) knots 0 0 0 1 2 2 2
  spline S60 degree 2 poles (-8.6001, -7.3894) (-8.6001, -7.54) (-8.4544, -7.75) (-8.3087, -7.834) knots 0 0 0 1 2 2 2
  spline S61 degree 2 poles (-8.3087, -7.834) (-8.2469, -7.8686) (-7.9851, -7.9896) (-7.8789, -8.0242) knots 0 0 0 1 2 2 2
  spline S62 degree 2 poles (-7.8789, -8.0242) (-7.7011, -7.8883) (-7.5751, -7.5993) (-7.5751, -7.4141) knots 0 0 0 1 2 2 2
  spline S63 degree 2 poles (-6.5864, -24.0878) (-6.5864, -24.9078) (-7.0631, -25.676) (-7.5596, -25.676) knots 0 0 0 1 2 2 2
  spline S64 degree 2 poles (-7.5596, -25.676) (-8.0635, -25.676) (-8.5353, -24.893) (-8.5353, -24.0902) knots 0 0 0 1 2 2 2
  spline S65 degree 2 poles (-8.5353, -24.0902) (-8.5353, -23.2653) (-8.0586, -22.502) (-7.5596, -22.502) knots 0 0 0 1 2 2 2
  spline S66 degree 2 poles (-7.5596, -22.502) (-7.0582, -22.502) (-6.5864, -23.2924) (-6.5864, -24.0878) knots 0 0 0 1 2 2 2
  spline S67 degree 2 poles (-7.1101, -25.0165) (-7.0508, -24.8658) (-7.0014, -24.4015) (-7.0014, -24.0878) knots 0 0 0 1 2 2 2
  spline S68 degree 2 poles (-7.0014, -24.0878) (-7.0014, -23.7741) (-7.0508, -23.3122) (-7.1125, -23.1566) knots 0 0 0 1 2 2 2
  spline S69 degree 2 poles (-7.1125, -23.1566) (-7.1743, -23.001) (-7.3892, -22.8404) (-7.5596, -22.8404) knots 0 0 0 1 2 2 2
  spline S70 degree 2 poles (-7.5596, -22.8404) (-7.73, -22.8404) (-7.9499, -23.001) (-8.0141, -23.1615) knots 0 0 0 1 2 2 2
  spline S71 degree 2 poles (-8.0141, -23.1615) (-8.0759, -23.3171) (-8.1203, -23.7914) (-8.1203, -24.0902) knots 0 0 0 1 2 2 2
  spline S72 degree 2 poles (-8.1203, -24.0902) (-8.1203, -24.4113) (-8.0808, -24.8411) (-8.0166, -25.0091) knots 0 0 0 1 2 2 2
  spline S73 degree 2 poles (-8.0166, -25.0091) (-7.9573, -25.1672) (-7.7375, -25.3376) (-7.5596, -25.3376) knots 0 0 0 1 2 2 2
  spline S74 degree 2 poles (-7.5596, -25.3376) (-7.3917, -25.3376) (-7.1718, -25.177) (-7.1101, -25.0165) knots 0 0 0 1 2 2 2
  spline S75 degree 2 poles (6.9477, -7.4859) (6.9477, -7.2513) (7.1009, -6.861) (7.2342, -6.7202) knots 0 0 0 1 2 2 2
  spline S76 degree 2 poles (7.2342, -6.7202) (7.3602, -6.5844) (7.7282, -6.4337) (7.916, -6.4337) knots 0 0 0 1 2 2 2
  spline S77 degree 2 poles (7.916, -6.4337) (8.1259, -6.4337) (8.4668, -6.5745) (8.5927, -6.7079) knots 0 0 0 1 2 2 2
  spline S78 degree 2 poles (8.5927, -6.7079) (8.7508, -6.8758) (8.9237, -7.4192) (8.9237, -7.8367) knots 0 0 0 1 2 2 2
  spline S79 degree 2 poles (8.9237, -7.8367) (8.9237, -8.2146) (8.7533, -8.8914) (8.5878, -9.1161) knots 0 0 0 1 2 2 2
  spline S80 degree 2 poles (8.5878, -9.1161) (8.4124, -9.3533) (7.9184, -9.6027) (7.5578, -9.6027) knots 0 0 0 1 2 2 2
  spline S81 degree 2 poles (7.5578, -9.6027) (7.4763, -9.6027) (7.291, -9.5854) (7.212, -9.5607) knots 0 0 0 1 2 2 2
  line L147 (7.212, -9.5607) -> (7.212, -9.168)
  line L148 (7.212, -9.168) -> (7.2318, -9.168)
  spline S82 degree 2 poles (7.2318, -9.168) (7.2836, -9.1976) (7.501, -9.2495) (7.6121, -9.2495) knots 0 0 0 1 2 2 2
  spline S83 degree 2 poles (7.6121, -9.2495) (8.0123, -9.2495) (8.4692, -8.7209) (8.5013, -8.2319) knots 0 0 0 1 2 2 2
  spline S84 degree 2 poles (8.5013, -8.2319) (8.3383, -8.343) (8.0419, -8.4443) (7.8666, -8.4443) knots 0 0 0 1 2 2 2
  spline S85 degree 2 poles (7.8666, -8.4443) (7.6986, -8.4443) (7.4195, -8.3702) (7.2787, -8.264) knots 0 0 0 1 2 2 2
  spline S86 degree 2 poles (7.2787, -8.264) (7.1157, -8.138) (6.9477, -7.7552) (6.9477, -7.4859) knots 0 0 0 1 2 2 2
  spline S87 degree 2 poles (8.5112, -7.7453) (8.5112, -7.4365) (8.3976, -7.0463) (8.2963, -6.94) knots 0 0 0 1 2 2 2
  spline S88 degree 2 poles (8.2963, -6.94) (8.2074, -6.8412) (8.0222, -6.7671) (7.9135, -6.7671) knots 0 0 0 1 2 2 2
  spline S89 degree 2 poles (7.9135, -6.7671) (7.6615, -6.7671) (7.3627, -7.1278) (7.3627, -7.4686) knots 0 0 0 1 2 2 2
  spline S90 degree 2 poles (7.3627, -7.4686) (7.3627, -7.6613) (7.4615, -7.9108) (7.5702, -7.9997) knots 0 0 0 1 2 2 2
  spline S91 degree 2 poles (7.5702, -7.9997) (7.6492, -8.0639) (7.8443, -8.1059) (7.9579, -8.1059) knots 0 0 0 1 2 2 2
  spline S92 degree 2 poles (7.9579, -8.1059) (8.0889, -8.1059) (8.3902, -8.0145) (8.5038, -7.9379) knots 0 0 0 1 2 2 2
  spline S93 degree 2 poles (8.5038, -7.9379) (8.5063, -7.9083) (8.5112, -7.807) (8.5112, -7.7453) knots 0 0 0 1 2 2 2
  spline S94 degree 2 poles (8.9125, 7.2482) (8.9125, 7.0135) (8.7569, 6.6159) (8.626, 6.4825) knots 0 0 0 1 2 2 2
  spline S95 degree 2 poles (8.626, 6.4825) (8.4902, 6.3417) (8.1493, 6.196) (7.9443, 6.196) knots 0 0 0 1 2 2 2
  spline S96 degree 2 poles (7.9443, 6.196) (7.7393, 6.196) (7.4009, 6.3343) (7.2724, 6.4726) knots 0 0 0 1 2 2 2
  spline S97 degree 2 poles (7.2724, 6.4726) (7.1144, 6.6381) (6.9365, 7.1939) (6.9365, 7.5989) knots 0 0 0 1 2 2 2
  spline S98 degree 2 poles (6.9365, 7.5989) (6.9365, 7.9966) (7.0995, 8.6363) (7.27, 8.8735) knots 0 0 0 1 2 2 2
  spline S99 degree 2 poles (7.27, 8.8735) (7.4355, 9.1057) (7.9591, 9.365) (8.3024, 9.365) knots 0 0 0 1 2 2 2
  spline S100 degree 2 poles (8.3024, 9.365) (8.4037, 9.365) (8.5815, 9.3452) (8.6482, 9.323) knots 0 0 0 1 2 2 2
  line L149 (8.6482, 9.323) -> (8.6482, 8.9303)
  line L150 (8.6482, 8.9303) -> (8.6309, 8.9303)
  spline S101 degree 2 poles (8.6309, 8.9303) (8.5741, 8.9599) (8.3667, 9.0118) (8.2481, 9.0118) knots 0 0 0 1 2 2 2
  spline S102 degree 2 poles (8.2481, 9.0118) (7.8677, 9.0118) (7.4009, 8.498) (7.3564, 7.9941) knots 0 0 0 1 2 2 2
  spline S103 degree 2 poles (7.3564, 7.9941) (7.5021, 8.0954) (7.8084, 8.2066) (7.9912, 8.2066) knots 0 0 0 1 2 2 2
  spline S104 degree 2 poles (7.9912, 8.2066) (8.1691, 8.2066) (8.4358, 8.1349) (8.5815, 8.0263) knots 0 0 0 1 2 2 2
  spline S105 degree 2 poles (8.5815, 8.0263) (8.7495, 7.9003) (8.9125, 7.51) (8.9125, 7.2482) knots 0 0 0 1 2 2 2
  spline S106 degree 2 poles (8.4976, 7.2309) (8.4976, 7.4186) (8.3988, 7.673) (8.2901, 7.762) knots 0 0 0 1 2 2 2
  spline S107 degree 2 poles (8.2901, 7.762) (8.2086, 7.8262) (8.006, 7.8682) (7.8998, 7.8682) knots 0 0 0 1 2 2 2
  spline S108 degree 2 poles (7.8998, 7.8682) (7.7566, 7.8682) (7.4873, 7.7817) (7.3564, 7.7002) knots 0 0 0 1 2 2 2
  spline S109 degree 2 poles (7.3564, 7.7002) (7.3539, 7.6558) (7.349, 7.5718) (7.349, 7.5076) knots 0 0 0 1 2 2 2
  spline S110 degree 2 poles (7.349, 7.5076) (7.349, 7.1914) (7.4725, 6.8036) (7.5664, 6.7023) knots 0 0 0 1 2 2 2
  spline S111 degree 2 poles (7.5664, 6.7023) (7.6528, 6.606) (7.8405, 6.5294) (7.9468, 6.5294) knots 0 0 0 1 2 2 2
  spline S112 degree 2 poles (7.9468, 6.5294) (8.1938, 6.5294) (8.4976, 6.8802) (8.4976, 7.2309) knots 0 0 0 1 2 2 2
  spline S113 degree 2 poles (25.1383, 7.1231) (25.1383, 6.8958) (24.9654, 6.5476) (24.8222, 6.4339) knots 0 0 0 1 2 2 2
  spline S114 degree 2 poles (24.8222, 6.4339) (24.6493, 6.3006) (24.2565, 6.1869) (23.9453, 6.1869) knots 0 0 0 1 2 2 2
  line L151 (23.9453, 6.1869) -> (23.0709, 6.1869)
  line L152 (23.0709, 6.1869) -> (23.0709, 9.2349)
  line L153 (23.0709, 9.2349) -> (23.8786, 9.2349)
  spline S115 degree 2 poles (23.8786, 9.2349) (24.2046, 9.2349) (24.5307, 9.1929) (24.6789, 9.1114) knots 0 0 0 1 2 2 2
  spline S116 degree 2 poles (24.6789, 9.1114) (24.8444, 9.025) (24.9951, 8.7409) (24.9951, 8.5483) knots 0 0 0 1 2 2 2
  spline S117 degree 2 poles (24.9951, 8.5483) (24.9951, 8.3334) (24.7678, 7.9925) (24.5677, 7.8962) knots 0 0 0 1 2 2 2
  line L154 (24.5677, 7.8962) -> (24.5677, 7.8814)
  spline S118 degree 2 poles (24.5677, 7.8814) (24.8394, 7.8073) (25.1383, 7.4145) (25.1383, 7.1231) knots 0 0 0 1 2 2 2
  spline S119 degree 2 poles (24.7159, 7.1058) (24.7159, 7.2787) (24.6171, 7.501) (24.4689, 7.58) knots 0 0 0 1 2 2 2
  spline S120 degree 2 poles (24.4689, 7.58) (24.3726, 7.6294) (24.1454, 7.6591) (23.9354, 7.6591) knots 0 0 0 1 2 2 2
  line L155 (23.9354, 7.6591) -> (23.476, 7.6591)
  line L156 (23.476, 7.6591) -> (23.476, 6.5327)
  line L157 (23.476, 6.5327) -> (23.8045, 6.5327)
  spline S121 degree 2 poles (23.8045, 6.5327) (24.0713, 6.5327) (24.3775, 6.5821) (24.4961, 6.6612) knots 0 0 0 1 2 2 2
  spline S122 degree 2 poles (24.4961, 6.6612) (24.6097, 6.7427) (24.7159, 6.9452) (24.7159, 7.1058) knots 0 0 0 1 2 2 2
  spline S123 degree 2 poles (24.5727, 8.4915) (24.5727, 8.6001) (24.4986, 8.7632) (24.4171, 8.8101) knots 0 0 0 1 2 2 2
  spline S124 degree 2 poles (24.4171, 8.8101) (24.3183, 8.8644) (24.0787, 8.8891) (23.8638, 8.8891) knots 0 0 0 1 2 2 2
  line L158 (23.8638, 8.8891) -> (23.476, 8.8891)
  line L159 (23.476, 8.8891) -> (23.476, 7.9975)
  line L160 (23.476, 7.9975) -> (23.9354, 7.9975)
  spline S125 degree 2 poles (23.9354, 7.9975) (24.1256, 7.9975) (24.3059, 8.037) (24.4022, 8.0987) knots 0 0 0 1 2 2 2
  spline S126 degree 2 poles (24.4022, 8.0987) (24.4961, 8.158) (24.5727, 8.3482) (24.5727, 8.4915) knots 0 0 0 1 2 2 2
  line L161 (9.2869, -23.4371) -> (8.6866, -23.4371)
  line L162 (8.6866, -23.4371) -> (8.5014, -24.2053)
  line L163 (8.5014, -24.2053) -> (9.0473, -24.2053)
  line L164 (9.0473, -24.2053) -> (9.0473, -24.4819)
  line L165 (9.0473, -24.4819) -> (8.4298, -24.4819)
  line L166 (8.4298, -24.4819) -> (8.2149, -25.344)
  line L167 (8.2149, -25.344) -> (7.9506, -25.344)
  line L168 (7.9506, -25.344) -> (8.1655, -24.4819)
  line L169 (8.1655, -24.4819) -> (7.6072, -24.4819)
  line L170 (7.6072, -24.4819) -> (7.3924, -25.344)
  line L171 (7.3924, -25.344) -> (7.1281, -25.344)
  line L172 (7.1281, -25.344) -> (7.343, -24.4819)
  line L173 (7.343, -24.4819) -> (6.8144, -24.4819)
  line L174 (6.8144, -24.4819) -> (6.8144, -24.2053)
  line L175 (6.8144, -24.2053) -> (7.4146, -24.2053)
  line L176 (7.4146, -24.2053) -> (7.5998, -23.4371)
  line L177 (7.5998, -23.4371) -> (7.054, -23.4371)
  line L178 (7.054, -23.4371) -> (7.054, -23.1605)
  line L179 (7.054, -23.1605) -> (7.6715, -23.1605)
  line L180 (7.6715, -23.1605) -> (7.8864, -22.296)
  line L181 (7.8864, -22.296) -> (8.1506, -22.296)
  line L182 (8.1506, -22.296) -> (7.9358, -23.1605)
  line L183 (7.9358, -23.1605) -> (8.494, -23.1605)
  line L184 (8.494, -23.1605) -> (8.7089, -22.296)
  line L185 (8.7089, -22.296) -> (8.9732, -22.296)
  line L186 (8.9732, -22.296) -> (8.7583, -23.1605)
  line L187 (8.7583, -23.1605) -> (9.2869, -23.1605)
  line L188 (9.2869, -23.1605) -> (9.2869, -23.4371)
  line L189 (8.4298, -23.4322) -> (7.8641, -23.4322)
  line L190 (7.8641, -23.4322) -> (7.6739, -24.2102)
  line L191 (7.6739, -24.2102) -> (8.2396, -24.2102)
  line L192 (8.2396, -24.2102) -> (8.4298, -23.4322)
  spline S127 degree 2 poles (25.084, -24.0285) (25.084, -24.4459) (24.7456, -25.1178) (24.4616, -25.3055) knots 0 0 0 1 2 2 2
  spline S128 degree 2 poles (24.4616, -25.3055) (24.2294, -25.4512) (23.7527, -25.55) (23.3822, -25.55) knots 0 0 0 1 2 2 2
  line L193 (23.3822, -25.55) -> (22.6807, -25.55)
  line L194 (22.6807, -25.55) -> (22.6807, -22.502)
  line L195 (22.6807, -22.502) -> (23.3748, -22.502)
  spline S129 degree 2 poles (23.3748, -22.502) (23.8046, -22.502) (24.2936, -22.6305) (24.4665, -22.7441) knots 0 0 0 1 2 2 2
  spline S130 degree 2 poles (24.4665, -22.7441) (24.7605, -22.9392) (25.084, -23.5839) (25.084, -24.0285) knots 0 0 0 1 2 2 2
  spline S131 degree 2 poles (24.6617, -24.0236) (24.6617, -23.6728) (24.4295, -23.1763) (24.1998, -23.0355) knots 0 0 0 1 2 2 2
  spline S132 degree 2 poles (24.1998, -23.0355) (24.0367, -22.9392) (23.6687, -22.8528) (23.3945, -22.8528) knots 0 0 0 1 2 2 2
  line L196 (23.3945, -22.8528) -> (23.0858, -22.8528)
  line L197 (23.0858, -22.8528) -> (23.0858, -25.1993)
  line L198 (23.0858, -25.1993) -> (23.3945, -25.1993)
  spline S133 degree 2 poles (23.3945, -25.1993) (23.6638, -25.1993) (24.0713, -25.1128) (24.2368, -24.9967) knots 0 0 0 1 2 2 2
  spline S134 degree 2 poles (24.2368, -24.9967) (24.4492, -24.8535) (24.6617, -24.3792) (24.6617, -24.0236) knots 0 0 0 1 2 2 2
  spline S135 degree 2 poles (23.8712, -9.1399) (23.5748, -9.1399) (23.0734, -8.9398) (22.8907, -8.7397) knots 0 0 0 1 2 2 2
  spline S136 degree 2 poles (22.8907, -8.7397) (22.7079, -8.5421) (22.5078, -7.9493) (22.5078, -7.564) knots 0 0 0 1 2 2 2
  spline S137 degree 2 poles (22.5078, -7.564) (22.5078, -7.1812) (22.7029, -6.6131) (22.8882, -6.4031) knots 0 0 0 1 2 2 2
  spline S138 degree 2 poles (22.8882, -6.4031) (23.071, -6.1981) (23.5699, -5.9832) (23.8787, -5.9832) knots 0 0 0 1 2 2 2
  spline S139 degree 2 poles (23.8787, -5.9832) (24.0318, -5.9832) (24.301, -6.0277) (24.4147, -6.0622) knots 0 0 0 1 2 2 2
  spline S140 degree 2 poles (24.4147, -6.0622) (24.5135, -6.0943) (24.7185, -6.1857) (24.8197, -6.2401) knots 0 0 0 1 2 2 2
  line L199 (24.8197, -6.2401) -> (24.8197, -6.7291)
  line L200 (24.8197, -6.7291) -> (24.7876, -6.7291)
  spline S141 degree 2 poles (24.7876, -6.7291) (24.7333, -6.6797) (24.5653, -6.5414) (24.4443, -6.4747) knots 0 0 0 1 2 2 2
  spline S142 degree 2 poles (24.4443, -6.4747) (24.3282, -6.4105) (24.054, -6.329) (23.8762, -6.329) knots 0 0 0 1 2 2 2
  spline S143 degree 2 poles (23.8762, -6.329) (23.6811, -6.329) (23.3328, -6.4895) (23.2019, -6.6427) knots 0 0 0 1 2 2 2
  spline S144 degree 2 poles (23.2019, -6.6427) (23.0734, -6.7983) (22.9302, -7.2701) (22.9302, -7.564) knots 0 0 0 1 2 2 2
  spline S145 degree 2 poles (22.9302, -7.564) (22.9302, -7.8777) (23.0808, -8.3297) (23.2118, -8.4853) knots 0 0 0 1 2 2 2
  spline S146 degree 2 poles (23.2118, -8.4853) (23.3402, -8.636) (23.6835, -8.7891) (23.8762, -8.7891) knots 0 0 0 1 2 2 2
  spline S147 degree 2 poles (23.8762, -8.7891) (24.0516, -8.7891) (24.3504, -8.7027) (24.4665, -8.6385) knots 0 0 0 1 2 2 2
  spline S148 degree 2 poles (24.4665, -8.6385) (24.5777, -8.5742) (24.7432, -8.4409) (24.7901, -8.3939) knots 0 0 0 1 2 2 2
  line L201 (24.7901, -8.3939) -> (24.8197, -8.3939)
  line L202 (24.8197, -8.3939) -> (24.8197, -8.8781)
  spline S149 degree 2 poles (24.8197, -8.8781) (24.7185, -8.925) (24.5406, -9.0114) (24.4147, -9.051) knots 0 0 0 1 2 2 2
  spline S150 degree 2 poles (24.4147, -9.051) (24.2813, -9.0954) (24.054, -9.1399) (23.8712, -9.1399) knots 0 0 0 1 2 2 2
  point P0 (0, 0)
  constraints: 32 other
extrude "Extrusion3" add sketch "Sketch4" along normal blind 0.2
body "Solid1"
